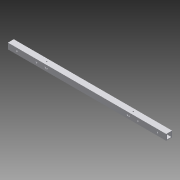
# Autodesk Inventor part: 1x1 horizontal lower
Saved by Autodesk Inventor 2015 SP1 (Build 190203100, 203)
## iProperties
Created: 2015-01-28
Part Number: 1x1 horizontal lower
Material: Aluminum 6061
Document SubType Name: Modeling
Designer: Admin
Density: 2.7 g/cm^3
Appearance: Aluminum - Flat
Author: Admin
Autodesk Inventor part; units mm, degrees
ref_plane "YZ Plane" through (0, 0, 0) normal (1, 0, 0) x (0, 1, 0)
ref_plane "XZ Plane" through (0, 0, 0) normal (0, 1, 0) x (-1, 0, 0)
ref_plane "XY Plane" through (0, 0, 0) normal (0, 0, 1) x (1, 0, 0)
sketch "Sketch1" plane through (0, 0, 0) normal (1, 0, 0) x (0, 1, 0)
  line L0 (0, 0) -> (25.4, 0)
  line L1 (25.4, 0) -> (25.4, -25.4)
  line L2 (25.4, -25.4) -> (0, -25.4)
  line L3 (0, -25.4) -> (0, 0)
  line L4 (3.175, -3.175) -> (22.225, -3.175)
  line L5 (22.225, -3.175) -> (22.225, -22.225)
  line L6 (22.225, -22.225) -> (3.175, -22.225)
  line L7 (3.175, -22.225) -> (3.175, -3.175)
  dimension "d0" = 25.4
  dimension "d1" = 25.4
  dimension "d2" = 19.05
  dimension "d3" = 19.05
  dimension "d4" = 3.175
  dimension "d5" = 3.175
  constraints: 16 end point, 4 parallel, 2 horizontal, 2 perpendicular
  measures "d0" distance of L1.end L2.end
  measures "d1" distance of L0.end L1.end
  measures "d2" distance of L5.end L6.end
  measures "d3" distance of L4.end L5.end
  measures "d4" distance between parallel lines of L0 L4
  measures "d5" distance between parallel lines of L3 L7
extrude "Extrusion1" add sketch "Sketch1" along normal blind 685.8
sketch "Sketch3" plane through (0, 0, -25.4) normal (0, 0, -1) x (-1, 0, 0)
  line L0 (0, 25.4) -> (0, 0) projected
  line L1 (-685.8, 0) -> (-685.8, 25.4) projected
  line L2 (0, 0) -> (-685.8, 0) projected
  point P0 (-647.7, 12.7)
  point P1 (-561.975, 12.7)
  point P2 (-523.875, 12.7)
  point P3 (-161.925, 12.7)
  point P4 (-123.825, 12.7)
  point P5 (-38.1, 12.7)
  dimension "d23" = 38.1
  dimension "d24" = 12.7
  dimension "d25" = 12.7
  dimension "d26" = 12.7
  dimension "d27" = 123.825
  dimension "d28" = 161.925
  dimension "d29" = 12.7
  dimension "d30" = 12.7
  dimension "d31" = 12.7
  dimension "d32" = 38.1
  dimension "d33" = 123.825
  dimension "d34" = 161.925
  measures "d23" distance from line of point (-647.7, 12.7) L1
  measures "d24" distance from line of L2 point (-647.7, 12.7)
  measures "d25" distance from line of L2 point (-561.975, 12.7)
  measures "d26" distance from line of L2 point (-523.875, 12.7)
  measures "d27" distance from line of L1 point (-561.975, 12.7)
  measures "d28" distance from line of L1 point (-523.875, 12.7)
  measures "d29" distance from line of L2 point (-38.1, 12.7)
  measures "d30" distance from line of L2 point (-123.825, 12.7)
  measures "d31" distance from line of L2 point (-161.925, 12.7)
  measures "d32" distance from line of L0 point (-38.1, 12.7)
  measures "d33" distance from line of point (-123.825, 12.7) L0
  measures "d34" distance from line of point (-161.925, 12.7) L0
hole "Hole2" at (647.7, 12.7, -25.4) at (561.975, 12.7, -25.4) at (523.875, 12.7, -25.4) at (161.925, 12.7, -25.4) at (123.825, 12.7, -25.4) at (38.1, 12.7, -25.4) direction (0, 0, 1) diameter 6.35 end through all
sketch "Sketch6" plane through (0, 0, -25.4) normal (0, 0, -1) x (-1, 0, 0)
  circle A0 centre (-523.875, 12.7) radius 3.175 projected
  circle A1 centre (-161.925, 12.7) radius 3.175 projected
  line L0 (0, 0) -> (-685.8, 0) projected
  circle A2 centre (-517.525, 12.7) radius 3.175
  circle A3 centre (-168.275, 12.7) radius 3.175
  dimension "d66" = 6.35
  dimension "d67" = 6.35
  dimension "d68" = 12.7
  dimension "d69" = 6.35
  dimension "d70" = 6.35
  dimension "d71" = 12.7
  constraints: 2 centre point
  measures "d66" diameter of A2
  measures "d67" diameter of A3
  measures "d68" distance from line of L0 A3.centre
  measures "d69" distance of A1.centre A3.centre
  measures "d70" distance of A0.centre A2.centre
  measures "d71" distance from line of L0 A2.centre
extrude "Extrusion2" cut sketch "Sketch6" against normal blind 25.4 contours A2 | A3
sketch "Sketch7" plane through (0, 25.4, 0) normal (0, 1, 0) x (1, 0, 0)
  line L0 (685.8, 25.4) -> (685.8, 0) projected
  line L1 (0, 25.4) -> (685.8, 25.4) projected
  point P0 (155.575, 12.7)
  point P1 (530.225, 12.7)
  dimension "d74" = 12.7
  dimension "d75" = 12.7
  dimension "d76" = 530.225
  dimension "d77" = 155.575
  measures "d74" distance from line of L1 point (155.575, 12.7)
  measures "d75" distance from line of L1 point (530.225, 12.7)
  measures "d76" distance from line of point (155.575, 12.7) L0
  measures "d77" distance from line of L0 point (530.225, 12.7)
hole "Hole5" at (155.575, 25.4, -12.7) at (530.225, 25.4, -12.7) direction (0, -1, 0) diameter 4.7625 depth 25.4 tip angle 118
body "Solid1"
